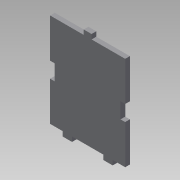
# Autodesk Inventor part: Bottom
Saved by Autodesk Inventor 2013 (Build 170138000, 138)
## iProperties
Created: 2013-12-12
Part Number: Bottom
Material: Generic
Document SubType Name: Modeling
Designer: Eric
Density: 1 g/cm^3
Author: Eric
Autodesk Inventor part; units mm, degrees
ref_plane "YZ Plane" through (0, 0, 0) normal (1, 0, 0) x (0, 1, 0)
ref_plane "XZ Plane" through (0, 0, 0) normal (0, 1, 0) x (-1, 0, 0)
ref_plane "XY Plane" through (0, 0, 0) normal (0, 0, 1) x (1, 0, 0)
sketch "Sketch1" plane through (0, 0, 0) normal (0, 1, 0) x (-1, 0, 0)
  line L0 (26.5, 66) -> (21.5, 66)
  line L1 (0, 63) -> (21.5, 63)
  line L2 (21.5, 63) -> (21.5, 66)
  line L3 (26.5, 66) -> (26.5, 63)
  line L4 (26.5, 63) -> (48, 63)
  line L5 (14, 0) -> (14, 3)
  line L6 (14, 3) -> (34, 3)
  line L7 (34, 3) -> (34, 0)
  line L8 (8, 0) -> (14, 0)
  line L9 (34, 0) -> (40, 0)
  line L10 (0, 63) -> (0, 38)
  line L11 (0, 28) -> (0, 3)
  line L12 (48, 3) -> (48, 28)
  line L13 (48, 38) -> (48, 63)
  line L14 (0, 38) -> (3, 38)
  line L15 (3, 38) -> (3, 28)
  line L16 (3, 28) -> (0, 28)
  line L17 (48, 38) -> (45, 38)
  line L18 (45, 38) -> (45, 28)
  line L19 (45, 28) -> (48, 28)
  line L20 (0, 3) -> (8, 3)
  line L21 (8, 3) -> (8, 0)
  line L22 (40, 3) -> (40, 0)
  line L23 (40, 3) -> (48, 3)
  point P0 (0, 0)
  dimension "d0" = 48
  dimension "d3" = 5
  dimension "d5" = 3
  dimension "d6" = 3
  dimension "d8" = 3
  dimension "d9" = 3
  dimension "d16" = 66
  dimension "d23" = 3
  dimension "d24" = 10
  dimension "d25" = 10
  dimension "d26" = 3
  dimension "d27" = 28
  dimension "d29" = 3
  dimension "d30" = 3
  dimension "d34" = 21.5
  dimension "d35" = 8
  dimension "d36" = 8
  dimension "d37" = 3
  dimension "d38" = 3
  dimension "d40" = 6
  dimension "d41" = 6
  dimension "d42" = 25
  dimension "d43" = 25
  constraints: 48 end point, 19 perpendicular, 10 parallel, 2 horizontal
  measures "d0" distance of L4.end L1.start
  measures "d3" distance of L0.start L0.end
  measures "d5" distance of L1.end L0.end
  measures "d6" distance of L0.start L3.end
  measures "d8" distance of L5.start L5.end
  measures "d9" distance of L6.end L7.end
  measures "d16" distance between parallel lines of L8 L0
  measures "d23" distance of L10.end L14.end
  measures "d24" distance of L14.end L15.end
  measures "d25" distance of L17.end L18.end
  measures "d26" distance of L13.start L17.end
  measures "d27" distance of L11.start point (0, 0)
  measures "d29" distance of L15.end L11.start
  measures "d30" distance of L18.end L12.end
  measures "d34" distance between parallel lines of L10 L2
  measures "d35" distance of L11.end L20.end
  measures "d36" distance of L22.start L12.start
  measures "d37" distance of L22.start L9.end
  measures "d38" distance of L20.end L8.start
  measures "d40" distance of L8.start L5.start
  measures "d41" distance of L7.end L9.end
  measures "d42" distance of L11.start L11.end
  measures "d43" distance of L12.start L12.end
extrude "Extrusion1" add sketch "Sketch1" along normal blind 3
body "Solid1"
